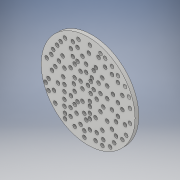
# Autodesk Inventor part: Part10
Saved by Autodesk Inventor 2017 (Build 210142000, 142)
## iProperties
Created: 2017-02-09
Part Number: Part10
Material: Generic
Document SubType Name: Modeling
Designer: XuZhiqing
Density: 1 g/cm^3
Appearance: Default
Author: XuZhiqing
Autodesk Inventor part; units mm, degrees
ref_plane "YZ Plane" through (0, 0, 0) normal (1, 0, 0) x (0, 1, 0)
ref_plane "XZ Plane" through (0, 0, 0) normal (0, 1, 0) x (-1, 0, 0)
ref_plane "XY Plane" through (0, 0, 0) normal (0, 0, 1) x (1, 0, 0)
sketch "Sketch1" plane through (0, 0, 0) normal (0, 0, 1) x (1, 0, 0)
  circle A0 centre (0, 0) radius 317.5
  circle A1 centre (-155.4707, 233.4453) radius 12.7
  circle A2 centre (-185.1298, 198.0458) radius 12.7
  circle A3 centre (-209.0484, 164.5598) radius 12.7
  circle A4 centre (-235.8372, 126.2901) radius 12.7
  circle A5 centre (-248.5372, 90.8906) radius 12.7
  circle A6 centre (-279.8473, 55.4911) radius 12.7
  circle A7 centre (-142.7707, 164.5598) radius 12.7
  circle A8 centre (-172.4298, 120.5496) radius 12.7
  circle A9 centre (-196.3484, 78.1906) radius 12.7
  circle A10 centre (-221.7484, 33.486) radius 12.7
  circle A11 centre (-243.4911, 0) radius 12.7
  circle A12 centre (-159.7298, 55.4911) radius 12.7
  circle A13 centre (-168.1707, 0) radius 12.7
  circle A14 centre (-159.7298, -41.14) radius 12.7
  circle A15 centre (-159.7298, -83.2366) radius 12.7
  circle A16 centre (-159.7298, -128.2036) radius 12.7
  circle A17 centre (-159.7298, -168.3868) radius 12.7
  circle A18 centre (-155.4707, -207.6132) radius 12.7
  circle A19 centre (5.2621, 225.7914) radius 12.7
  circle A20 centre (-37.7914, 185.3458) radius 12.7
  circle A21 centre (-71.2774, 138.9901) radius 12.7
  circle A22 centre (-90.4122, 113.5901) radius 12.7
  circle A23 centre (-118.1578, 78.1906) radius 12.7
  circle A24 centre (53.0992, 164.5598) radius 12.7
  circle A25 centre (96.1527, 126.2901) radius 12.7
  circle A26 centre (129.6387, 95.6743) radius 12.7
  circle A27 centre (168.8651, 65.4906) radius 12.7
  circle A28 centre (202.3512, 33.486) radius 12.7
  circle A29 centre (232.0102, 7.6539) radius 12.7
  circle A30 centre (-50.4914, 90.8906) radius 12.7
  circle A31 centre (-12.916, 103.5906) radius 12.7
  circle A32 centre (25.3537, 90.8906) radius 12.7
  circle A33 centre (71.2774, 82.9743) radius 12.7
  circle A34 centre (-90.4122, 33.486) radius 12.7
  circle A35 centre (-50.4914, 33.486) radius 12.7
  circle A36 centre (-0.216, 33.486) radius 12.7
  circle A37 centre (38.0537, 27.7455) radius 12.7
  circle A38 centre (83.9774, 27.7455) radius 12.7
  circle A39 centre (129.6387, 20.786) radius 12.7
  circle A40 centre (17.9621, 65.4906) radius 12.7
  circle A41 centre (17.9621, -5.0461) radius 12.7
  circle A42 centre (12.484, -53.84) radius 12.7
  circle A43 centre (12.484, -83.2366) radius 12.7
  circle A44 centre (12.484, -123.4199) radius 12.7
  circle A45 centre (12.484, -155.6868) radius 12.7
  circle A46 centre (12.484, -220.3132) radius 12.7
  circle A47 centre (-25.616, -244.9262) radius 12.7
  circle A48 centre (-50.4914, -220.3132) radius 12.7
  circle A49 centre (-77.7122, -168.3868) radius 12.7
  circle A50 centre (-37.7914, -78.4529) radius 12.7
  circle A51 centre (-90.4122, -123.4199) radius 12.7
  circle A52 centre (83.9774, -78.4529) radius 12.7
  circle A53 centre (129.6387, -110.7199) radius 12.7
  circle A54 centre (162.1679, -142.9868) radius 12.7
  circle A55 centre (189.6512, -168.3868) radius 12.7
  circle A56 centre (50.7537, -130.2868) radius 12.7
  circle A57 centre (96.6774, -181.0868) radius 12.7
  circle A58 centre (102.8499, -233.0132) radius 12.7
  circle A59 centre (50.7537, -265.0178) radius 12.7
  circle A60 centre (-25.0914, -283.196) radius 12.7
  circle A61 centre (-90.4122, -252.3178) radius 12.7
  circle A62 centre (-155.4707, -239.6178) radius 12.7
  circle A63 centre (-221.7484, -181.0868) radius 12.7
  circle A64 centre (-230.7911, -110.7199) radius 12.7
  circle A65 centre (-203.3079, -53.84) radius 12.7
  circle A66 centre (-267.1473, -59.3181) radius 12.7
  circle A67 centre (-286.5445, -91.1529) radius 12.7
  circle A68 centre (-267.1473, -130.2868) radius 12.7
  circle A69 centre (-103.1122, 151.8598) radius 12.7
  circle A70 centre (-103.1122, 238.4914) radius 12.7
  circle A71 centre (-65.0122, 270.7583) radius 12.7
  circle A72 centre (-71.2774, 220.7453) radius 12.7
  circle A73 centre (-115.8122, 191.3486) radius 12.7
  circle A74 centre (71.2774, 233.4453) radius 12.7
  circle A75 centre (115.5499, 198.0458) radius 12.7
  circle A76 centre (162.1679, 178.6486) radius 12.7
  circle A77 centre (202.3512, 151.8598) radius 12.7
  circle A78 centre (232.0102, 90.8906) radius 12.7
  circle A79 centre (283.6743, 40.4455) radius 12.7
  circle A80 centre (162.1679, -28.44) radius 12.7
  circle A81 centre (250.1883, -72.0181) radius 12.7
  circle A82 centre (189.6512, -84.7181) radius 12.7
  circle A83 centre (102.8499, -41.14) radius 12.7
  circle A84 centre (58.5774, -17.7461) radius 12.7
  circle A85 centre (202.3512, -46.6181) radius 12.7
  circle A86 centre (283.6743, -46.6181) radius 12.7
  circle A87 centre (257.8422, -130.2868) radius 12.7
  circle A88 centre (232.0102, -168.3868) radius 12.7
  circle A89 centre (176.9512, -214.3105) radius 12.7
  circle A90 centre (149.4679, -252.3178) radius 12.7
  circle A91 centre (96.6774, -270.496) radius 12.7
  circle A92 centre (58.5774, -214.3105) radius 12.7
  circle A93 centre (-12.3914, -175.084) radius 12.7
  circle A94 centre (-71.2774, -97.4181) radius 12.7
  circle A95 centre (-90.4122, -46.6181) radius 12.7
  circle A96 centre (-37.7914, -5.0461) radius 12.7
  circle A97 centre (-96.1527, -5.0461) radius 12.7
  circle A98 centre (-115.8122, -84.7181) radius 12.7
  circle A99 centre (-118.1578, -155.6868) radius 12.7
  circle A100 centre (-118.1578, -207.6132) radius 12.7
  circle A101 centre (-25.616, -142.9868) radius 12.7
  circle A102 centre (-12.916, 151.8598) radius 12.7
  circle A103 centre (38.0537, 139.1598) radius 12.7
  circle A104 centre (12.484, 275.542) radius 12.7
  circle A105 centre (83.9774, 262.842) radius 12.7
  circle A106 centre (115.5499, 250.142) radius 12.7
  circle A107 centre (162.1679, 225.7914) radius 12.7
  circle A108 centre (202.3512, 191.3486) radius 12.7
  circle A109 centre (250.1883, 151.8598) radius 12.7
  circle A110 centre (276.9771, 103.5906) radius 12.7
  dimension "d0" = 635
  dimension "d1" = 25.4
  dimension "d2" = 25.4
  dimension "d3" = 25.4
  dimension "d4" = 25.4
  dimension "d5" = 25.4
  dimension "d6" = 25.4
  dimension "d7" = 25.4
  dimension "d8" = 25.4
  dimension "d9" = 25.4
  dimension "d10" = 25.4
  dimension "d11" = 25.4
  dimension "d12" = 25.4
  dimension "d13" = 25.4
  dimension "d14" = 25.4
  dimension "d15" = 25.4
  dimension "d16" = 25.4
  dimension "d17" = 25.4
  dimension "d18" = 25.4
  dimension "d19" = 25.4
  dimension "d20" = 25.4
  dimension "d21" = 25.4
  dimension "d22" = 25.4
  dimension "d23" = 25.4
  dimension "d25" = 25.4
  dimension "d26" = 25.4
  dimension "d27" = 25.4
  dimension "d28" = 25.4
  dimension "d29" = 25.4
  dimension "d30" = 25.4
  dimension "d31" = 25.4
  dimension "d32" = 25.4
  dimension "d33" = 25.4
  dimension "d34" = 25.4
  dimension "d35" = 25.4
  dimension "d36" = 25.4
  dimension "d37" = 25.4
  dimension "d38" = 25.4
  dimension "d39" = 25.4
  dimension "d40" = 25.4
  dimension "d41" = 25.4
  dimension "d42" = 25.4
  dimension "d43" = 25.4
  dimension "d44" = 25.4
  dimension "d45" = 25.4
  dimension "d46" = 25.4
  dimension "d48" = 25.4
  dimension "d49" = 25.4
  dimension "d50" = 25.4
  dimension "d51" = 25.4
  dimension "d52" = 25.4
  dimension "d54" = 25.4
  dimension "d55" = 25.4
  dimension "d56" = 25.4
  dimension "d57" = 25.4
  dimension "d58" = 25.4
  dimension "d59" = 25.4
  dimension "d60" = 25.4
  dimension "d61" = 25.4
  dimension "d62" = 25.4
  dimension "d63" = 25.4
  dimension "d64" = 25.4
  dimension "d65" = 25.4
  dimension "d66" = 25.4
  constraints: 111 centre point, 1 coincident
  measures "d0" diameter of A0
  measures "d1" diameter of A1
  measures "d2" diameter of A2
  measures "d3" diameter of A3
  measures "d4" diameter of A4
  measures "d5" diameter of A5
  measures "d6" diameter of A6
  measures "d7" diameter of A7
  measures "d8" diameter of A8
  measures "d9" diameter of A9
  measures "d10" diameter of A10
  measures "d11" diameter of A11
  measures "d12" diameter of A12
  measures "d13" diameter of A13
  measures "d14" diameter of A14
  measures "d15" diameter of A15
  measures "d16" diameter of A16
  measures "d17" diameter of A17
  measures "d18" diameter of A18
  measures "d19" diameter of A19
  measures "d20" diameter of A20
  measures "d21" diameter of A21
  measures "d22" diameter of A22
  measures "d23" diameter of A23
  measures "d25" diameter of A24
  measures "d26" diameter of A25
  measures "d27" diameter of A26
  measures "d28" diameter of A27
  measures "d29" diameter of A28
  measures "d30" diameter of A29
  measures "d31" diameter of A30
  measures "d32" diameter of A31
  measures "d33" diameter of A32
  measures "d34" diameter of A33
  measures "d35" diameter of A34
  measures "d36" diameter of A35
  measures "d37" diameter of A36
  measures "d38" diameter of A37
  measures "d39" diameter of A38
  measures "d40" diameter of A39
  measures "d41" diameter of A40
  measures "d42" diameter of A41
  measures "d43" diameter of A42
  measures "d44" diameter of A43
  measures "d45" diameter of A44
  measures "d46" diameter of A45
  measures "d48" diameter of A46
  measures "d49" diameter of A47
  measures "d50" diameter of A48
  measures "d51" diameter of A49
  measures "d52" diameter of A50
  measures "d54" diameter of A51
  measures "d55" diameter of A52
  measures "d56" diameter of A53
  measures "d57" diameter of A54
  measures "d58" diameter of A55
  measures "d59" diameter of A56
  measures "d60" diameter of A57
  measures "d61" diameter of A58
  measures "d62" diameter of A59
  measures "d63" diameter of A60
  measures "d64" diameter of A61
  measures "d65" diameter of A62
  measures "d66" diameter of A63
extrude "Extrusion1" add sketch "Sketch1" along normal blind 25.4 contours A0 | A7
body "Solid1"
